Nut 8 (Autodesk Fusion 360 design; units mm, degrees)
Autodesk Fusion 360 part; units mm, degrees
sketch "Sketch1" plane through (0, 0, 0) normal (0, 0, 1) x (1, 0, 0)
  circle A0 centre (0, 0) radius 4
  line L0 (0, -7.5056) -> (6.5, -3.7528)
  line L1 (6.5, -3.7528) -> (6.5, 3.7528)
  line L2 (6.5, 3.7528) -> (0, 7.5056)
  line L3 (0, 7.5056) -> (-6.5, 3.7528)
  line L4 (-6.5, 3.7528) -> (-6.5, -3.7528)
  line L5 (-6.5, -3.7528) -> (0, -7.5056)
  dimension "d1" = 8
  dimension "d2" = 13
  constraint coincident A0.centre origin
  measures "d1" diameter of A0
  measures "d2" distance of L0 L3
extrude "Extrude1" add sketch "Sketch1" along normal blind 3.5
fillet "Fillet1" radius 0.5 20 edges at (-3.7293, 1.4465, 0) (-6.5, -3.7528, 1.75) (3.25, 5.6292, 0) (-3.25, 5.6292, 3.5) (3.25, -5.6292, 3.5) (6.5, 3.7528, 1.75) (6.5, 0, 0) (-6.5, 0, 0) (-6.5, 3.7528, 1.75) (6.5, -3.7528, 1.75) (-3.25, -5.6292, 3.5) (-6.5, 0, 3.5) (3.25, -5.6292, 0) (-3.25, -5.6292, 0) (-3.7293, 1.4465, 3.5) (0, 7.5056, 1.75) (0, -7.5056, 1.75) (3.25, 5.6292, 3.5) (6.5, 0, 3.5) (-3.25, 5.6292, 0) 9 faces at (-6.5, 1.2509, 1.1667) (6.5, -1.2509, 1.1667) (-2.1667, 6.2546, 1.1667) (2.1667, -6.2546, 1.1667) (3.9801, -0.3983, 2.3333) (-4.3333, -5.0037, 1.1667) (5.6667, 0, 3.5) (5.6667, 0, 0) (4.3333, 5.0037, 1.1667)
